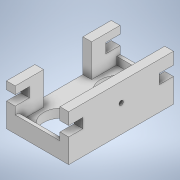
# Autodesk Inventor part: Ultrasound Mount 4
Saved by Autodesk Inventor 2020 (Build 240168000, 168)
## iProperties
Created: 2019-07-31
Part Number: Ultrasound Mount 4
Material: Generic
Document SubType Name: Modeling
Designer: cui_t
Density: 1 g/cm^3
Appearance: Default
Author: cui_t
Autodesk Inventor part; units mm, degrees
ref_plane "YZ Plane" through (0, 0, 0) normal (1, 0, 0) x (0, 1, 0)
ref_plane "XZ Plane" through (0, 0, 0) normal (0, 1, 0) x (-1, 0, 0)
ref_plane "XY Plane" through (0, 0, 0) normal (0, 0, 1) x (1, 0, 0)
sketch "Sketch1" plane through (0, 0, 0) normal (0, 1, 0) x (-1, 0, 0)
  line L0 (14.25, 24) -> (-14.25, 24)
  line L1 (-14.25, 24) -> (-14.25, -24)
  line L2 (-14.25, -24) -> (14.25, -24)
  line L3 (14.25, -24) -> (14.25, 24)
  line L4 (14.25, 24) -> (-14.25, -24) construction
  line L5 (-14.25, 24) -> (14.25, -24) construction
  point P0 (0, 0)
  dimension "d0" = 28.5
  dimension "d1" = 48
  constraints: 12 end point, 2 midpoint, 2 parallel, 1 horizontal, 1 perpendicular
  measures "d0" distance of L2.end L1.end
  measures "d1" distance of L0.end L1.end
extrude "Extrusion1" add sketch "Sketch1" along normal blind 4
sketch "Sketch2" plane through (0, 4, 0) normal (0, 1, 0) x (1, 0, 0)
  circle A0 centre (0, -13) radius 8.25
  circle A1 centre (0, 13) radius 8.25
  line L0 (14.25, 24) -> (-14.25, 24) projected
  line L1 (-14.25, 24) -> (-14.25, -24) projected
  point P0 (0, 0)
  dimension "d4" = 16.5
  dimension "d5" = 16.5
  dimension "d6" = 26
  dimension "d7" = 11
  dimension "d8" = 14.25
  dimension "d9" = 14.25
  constraints: 2 centre point
  measures "d4" diameter of A0
  measures "d5" diameter of A1
  measures "d6" distance of A0.centre A1.centre
  measures "d7" distance from line of L0 A1.centre
  measures "d8" distance from line of L1 A1.centre
  measures "d9" distance from line of L1 A0.centre
extrude "Extrusion2" cut sketch "Sketch2" against normal blind 4
sketch "Sketch3" plane through (0, 4, 0) normal (0, 1, 0) x (1, 0, 0)
  line L0 (14.25, -24) -> (10.25, -24)
  line L1 (10.25, -24) -> (10.25, 24)
  line L2 (10.25, 24) -> (14.25, 24)
  line L3 (14.25, 24) -> (14.25, -24)
  line L4 (14.25, -24) -> (10.25, 24) construction
  line L5 (10.25, -24) -> (14.25, 24) construction
  line L6 (14.25, -24) -> (14.25, 24) projected
  line L7 (14.25, 24) -> (-14.25, 24) projected
  point P0 (0, 0)
  point P1 (12.25, 0)
  dimension "d12" = 48
  dimension "d13" = 4
  constraints: 12 end point, 2 collinear, 2 midpoint, 2 parallel, 1 horizontal, 1 perpendicular
  measures "d12" distance of L2.end L0.start
  measures "d13" distance of L1.end L2.end
extrude "Extrusion3" add sketch "Sketch3" along normal blind 17
sketch "Sketch4" plane through (0, 4, 0) normal (0, 1, 0) x (1, 0, 0)
  line L0 (-14.25, -24) -> (-10.25, -24)
  line L1 (-10.25, -24) -> (-10.25, -11)
  line L2 (-10.25, -11) -> (-14.25, -11)
  line L3 (-14.25, -11) -> (-14.25, -24)
  line L4 (-14.25, -24) -> (10.25, -24) projected
  line L5 (-14.25, 24) -> (-14.25, -24) projected
  line L6 (-14.25, 24) -> (-10.25, 24)
  line L7 (-10.25, 24) -> (-10.25, 11)
  line L8 (-10.25, 11) -> (-14.25, 11)
  line L9 (-14.25, 11) -> (-14.25, 24)
  point P0 (0, 0)
  dimension "d16" = 4
  dimension "d17" = 13
  dimension "d18" = 4
  dimension "d19" = 13
  constraints: 16 end point, 4 parallel, 2 collinear, 2 horizontal, 2 perpendicular
  measures "d16" distance of L2.end L1.end
  measures "d17" distance of L1.end L0.end
  measures "d18" distance of L7.end L8.end
  measures "d19" distance of L6.end L7.end
extrude "Extrusion4" add sketch "Sketch4" along normal blind 15
sketch "Sketch5" plane through (-14.25, 0, -24) normal (-1, 0, 0) x (0, 0, 1)
  line L0 (41.5, 15.5) -> (48, 15.5)
  line L1 (48, 15.5) -> (48, 11)
  line L2 (48, 11) -> (41.5, 11)
  line L3 (41.5, 11) -> (41.5, 15.5)
  line L4 (35, 4) -> (35, 19) projected
  line L5 (0, 0) -> (48, 0) projected
  line L6 (0, 15.5) -> (6.5, 15.5)
  line L7 (6.5, 15.5) -> (6.5, 11)
  line L8 (6.5, 11) -> (0, 11)
  line L9 (0, 11) -> (0, 15.5)
  line L10 (13, 4) -> (13, 19) projected
  line L11 (48, 0) -> (48, 19) projected
  line L12 (0, 0) -> (0, 19) projected
  point P0 (24, 0)
  dimension "d22" = 6.5
  dimension "d23" = 4.5
  dimension "d24" = 11
  dimension "d25" = 6.5
  dimension "d26" = 4.5
  dimension "d27" = 11
  constraints: 16 end point, 2 collinear, 2 horizontal, 2 parallel, 1 perpendicular
  measures "d22" distance of L1.end L2.end
  measures "d23" distance of L0.end L1.end
  measures "d24" distance between parallel lines of L5 L2
  measures "d25" distance of L7.end L8.end
  measures "d26" distance of L6.end L7.end
  measures "d27" distance between parallel lines of L5 L8
extrude "Extrusion5" cut sketch "Sketch5" against normal blind 4
sketch "Sketch6" plane through (10.25, 4, -24) normal (-1, 0, 0) x (0, 0, 1)
  point P0 (24, -4)
sketch "Sketch7" plane through (10.25, 4, -24) normal (-1, 0, 0) x (0, 0, 1)
  circle A0 centre (24, 8.5) radius 2.625
  line L0 (13, 0) -> (35, 0) projected
  point P0 (24, -4)
  dimension "d30" = 5.25
  dimension "d31" = 8.5
  constraints: 1 centre point
  measures "d30" diameter of A0
  measures "d31" distance from line of L0 A0.centre
extrude "Extrusion6" cut sketch "Sketch7" against normal blind 2
sketch "Sketch8" plane through (12.25, 12.5, 0) normal (-1, 0, 0) x (0, 0, 1)
  circle A0 centre (0, 0) radius 2.625 projected
  circle A1 centre (0, 0) radius 1
  point P0 (0, -12.5)
  dimension "d34" = 2
  constraints: 1 centre point, 1 coincident
  measures "d34" diameter of A1
extrude "Extrusion7" cut sketch "Sketch8" against normal blind 2 contours A1
sketch "Sketch9" plane through (0, 4, 0) normal (0, 1, 0) x (1, 0, 0)
  line L0 (-10.25, -24) -> (10.25, -24)
  line L1 (10.25, -24) -> (10.25, -22.5)
  line L2 (10.25, -22.5) -> (-10.25, -22.5)
  line L3 (-10.25, -22.5) -> (-10.25, -24)
  line L4 (-10.25, -11) -> (-10.25, -24) projected
  line L5 (-10.25, -24) -> (10.25, -24) projected
  line L6 (-10.25, 22.5) -> (10.25, 22.5)
  line L7 (10.25, 22.5) -> (10.25, 24)
  line L8 (10.25, 24) -> (-10.25, 24)
  line L9 (-10.25, 24) -> (-10.25, 22.5)
  line L10 (-10.25, 24) -> (-10.25, 11) projected
  line L11 (10.25, 24) -> (-10.25, 24) projected
  point P0 (0, 0)
  dimension "d37" = 20.5
  dimension "d38" = 1.5
  dimension "d39" = 1.5
  dimension "d40" = 20.5
  constraints: 16 end point, 4 collinear, 4 parallel, 2 horizontal, 2 perpendicular
  measures "d37" distance of L1.end L2.end
  measures "d38" distance of L0.end L1.end
  measures "d39" distance of L6.end L7.end
  measures "d40" distance of L7.end L8.end
extrude "Extrusion8" add sketch "Sketch9" along normal blind 3.5
sketch "Sketch10" plane through (14.25, 0, 24) normal (1, 0, 0) x (0, 0, -1)
  line L0 (48, 15.5) -> (41.5, 15.5)
  line L1 (41.5, 15.5) -> (41.5, 11)
  line L2 (41.5, 11) -> (48, 11)
  line L3 (48, 11) -> (48, 15.5)
  line L4 (41.5, 11) -> (41.5, 15.5) projected
  line L5 (41.5, 15.5) -> (48, 15.5) projected
  line L6 (48, 0) -> (48, 21) projected
  line L7 (0, 0) -> (48, 0) projected
  point P0 (24, 0)
  dimension "d43" = 4.5
  dimension "d44" = 6.5
  dimension "d45" = 11
  constraints: 8 end point, 4 equal length, 1 collinear, 1 horizontal, 1 perpendicular
  measures "d43" distance of L0.end L1.end
  measures "d44" distance of L1.end L2.end
  measures "d45" distance between parallel lines of L7 L2
sketch "Sketch11" plane through (14.25, 0, 24) normal (1, 0, 0) x (0, 0, -1)
  line L0 (6.5, 15.5) -> (0, 15.5)
  line L1 (0, 15.5) -> (0, 11)
  line L2 (0, 11) -> (6.5, 11)
  line L3 (6.5, 11) -> (6.5, 15.5)
  line L4 (0, 0) -> (48, 0) projected
  line L5 (0, 0) -> (0, 21) projected
  point P0 (24, 0)
  dimension "d46" = 6.5
  dimension "d47" = 4.5
  dimension "d48" = 11
  constraints: 8 end point, 2 parallel, 1 collinear, 1 horizontal, 1 perpendicular
  measures "d46" distance of L2.end L1.end
  measures "d47" distance of L0.end L1.end
  measures "d48" distance between parallel lines of L4 L2
extrude "Extrusion9" cut sketch "Sketch10" against normal blind 4
extrude "Extrusion10" cut sketch "Sketch11" against normal blind 4
body "Solid1"
